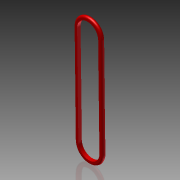
# Autodesk Inventor part: 7in polycord loop
Saved by Autodesk Inventor 2011 SP1 (Build 150282100, 282)
## iProperties
Created: 2012-01-20
Part Number: 7in polycord loop
Document SubType Name: Modeling
Designer: Christopher
Density: 1 g/cm^3
Author: Christopher
Autodesk Inventor part; units mm, degrees
ref_plane "YZ Plane" through (0, 0, 0) normal (1, 0, 0) x (0, 1, 0)
ref_plane "XZ Plane" through (0, 0, 0) normal (0, 1, 0) x (-1, 0, 0)
ref_plane "XY Plane" through (0, 0, 0) normal (0, 0, 1) x (1, 0, 0)
sketch "Sketch1" plane through (0, 0, 0) normal (0, 0, 1) x (1, 0, 0)
  line L0 (25.7585, 0.0668) -> (23.5051, 178.1043)
  line L1 (-24.7511, 177.4935) -> (-22.4976, -0.544)
  line L2 (32.1011, 0.692) -> (29.8546, 178.1847)
  line L3 (-31.1006, 177.4131) -> (-28.854, -0.0795)
  arc A0 (29.8546, 178.1847) -> (-31.1006, 177.4131) centre (-0.623, 177.7989) ccw
  arc A1 (-28.854, -0.0795) -> (32.1011, 0.692) centre (1.6236, 0.3063) ccw
  arc A2 (-22.4976, -0.544) -> (25.7585, 0.0668) centre (1.6305, -0.2386) ccw
  arc A3 (23.5051, 178.1043) -> (-24.7511, 177.4935) centre (-0.623, 177.7989) ccw
  point P0 (0, 0)
  dimension "d6" = 6.35
  dimension "d7" = 6.35
  dimension "d11" = 177.8
  dimension "d12" = 177.8
  dimension "d13" = 24.13
  constraints: 8 end point, 8 point on circle, 4 centre point, 4 tangent, 2 parallel, 1 coincident
  measures "d6" distance between parallel lines of L1 L3
  measures "d7" distance between parallel lines of L2 L0
  measures "d11" distance of A0.centre point (0, 0)
  measures "d12" distance of point (0, 0) A3.centre
  measures "d13" distance from line of A0.centre L0
extrude "Extrusion1" add sketch "Sketch1" against normal blind 6.35
fillet "Fillet1" radius 3.175 8 edges at (30.9778, 89.4384, 0) (-1.0088, 208.2765, 0) (-29.9773, 88.6668, 0) (2.0093, -30.1713, 0) (30.9778, 89.4384, -6.35) (-1.0088, 208.2765, -6.35) (-29.9773, 88.6668, -6.35) (2.0093, -30.1713, -6.35)
body "Solid1"
